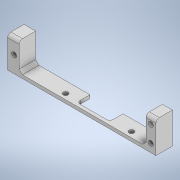
# Autodesk Inventor part: atx-adapter_mount
Saved by Autodesk Inventor 2021 (Build 250183000, 183)
## iProperties
Created: 2024-03-17
Part Number: atx-adapter_mount
Material: Generic
Document SubType Name: Modeling
Designer: Toby
Density: 1 g/cm^3
Appearance: Default
Author: Toby
Autodesk Inventor part; units mm, degrees
ref_plane "YZ Plane" through (0, 0, 0) normal (1, 0, 0) x (0, 1, 0)
ref_plane "XZ Plane" through (0, 0, 0) normal (0, 1, 0) x (-1, 0, 0)
ref_plane "XY Plane" through (0, 0, 0) normal (0, 0, 1) x (1, 0, 0)
sketch "Sketch1" plane through (0, 0, 0) normal (0, 0, 1) x (1, 0, 0)
  line L0 (-40.9154, -1.8235) -> (49.0846, -1.8235)
  line L1 (49.0846, -1.8235) -> (49.0846, -3.8235)
  line L2 (49.0846, -3.8235) -> (-40.9154, -3.8235)
  line L3 (-40.9154, -3.8235) -> (-40.9154, -1.8235)
  line L4 (-40.9154, -1.8235) -> (-33.9154, -1.8235)
  line L5 (-33.9154, -1.8235) -> (-33.9154, 15.1765)
  line L6 (-33.9154, 15.1765) -> (-40.9154, 15.1765)
  line L7 (-40.9154, 15.1765) -> (-40.9154, -1.8235)
  line L8 (49.0846, -1.8235) -> (43.0846, -1.8235)
  line L9 (43.0846, -1.8235) -> (43.0846, 15.1765)
  line L10 (43.0846, 15.1765) -> (49.0846, 15.1765)
  line L11 (49.0846, 15.1765) -> (49.0846, -1.8235)
  circle A0 centre (-36.9154, 6.1765) radius 1.5
  circle A1 centre (46.0846, 11.1765) radius 1.5
  circle A2 centre (46.0846, 1.1765) radius 1.5
  point P0 (0, 0)
  point P1 (43.0846, -1.8235)
  point P2 (43.0846, -1.8235)
  dimension "d0" = 2
  dimension "d1" = 90
  dimension "d2" = 10
  dimension "d3" = 5
  dimension "d4" = 15
  dimension "d5" = 83
  dimension "d6" = 83
  dimension "d7" = 4
  dimension "d8" = 3
  dimension "d9" = 3
  dimension "d10" = 3
  dimension "d11" = 19
  dimension "d12" = 3
  dimension "d13" = 3
  dimension "d14" = 3
  constraints: 24 end point, 6 parallel, 3 centre point, 3 coincident, 3 horizontal, 3 perpendicular, 1 point on line
  measures "d0" distance between parallel lines of L2 L0
  measures "d1" distance of L0.start L0.end
  measures "d2" distance from line of L2 point (-36.915, 6.177)
  measures "d3" distance from line of L2 point (46.085, 1.177)
  measures "d4" distance from line of L2 point (46.085, 11.177)
  measures "d5" horizontal distance of point (-36.915, 6.177) point (46.085, 11.177)
  measures "d6" horizontal distance of point (-36.915, 6.177) point (46.085, 1.177)
  measures "d7" distance from line of L7 point (-36.915, 6.177)
  measures "d8" distance from line of point (-36.915, 6.177) L5
  measures "d9" distance from line of point (46.085, 1.177) L9
  measures "d10" distance from line of point (46.085, 1.177) L11
  measures "d11" distance between parallel lines of L2 L10
  measures "d12" diameter of A0
  measures "d13" diameter of A1
  measures "d14" diameter of A2
extrude "Extrusion1" add sketch "Sketch1" against normal blind 10 contours L7 L6 L5 L0 | L0 L1 L2 L3 | L9 L10 L11 L0 | A0 | A1 | A2
fillet "Fillet1" radius 2 2 edges at (-37.4154, 15.1765, 0) (46.0846, 15.1765, 0)
sketch "Sketch2" plane through (0, 0, 0) normal (0, 0, 1) x (1, 0, 0)
  line L0 (-40.9154, -3.8235) -> (49.0846, -3.8235) projected
  line L1 (-40.9154, 13.1765) -> (-40.9154, -3.8235) projected
  line L2 (49.0846, -3.8235) -> (49.0846, 13.1765) projected
  point P0 (0, 0)
  point P1 (-36.9154, 6.1765)
  point P2 (46.0846, 1.1765)
  point P3 (46.0846, 11.1765)
  dimension "d18" = 10
  dimension "d19" = 5
  dimension "d20" = 15
  dimension "d21" = 4
  dimension "d22" = 83
  dimension "d23" = 83
  dimension "d24" = 3
  measures "d18" distance from line of L0 point (-36.915, 6.177)
  measures "d19" distance from line of L0 point (46.085, 1.177)
  measures "d20" distance from line of L0 point (46.085, 11.177)
  measures "d21" distance from line of L1 point (-36.915, 6.177)
  measures "d22" horizontal distance of point (46.085, 11.177) point (-36.915, 6.177)
  measures "d23" horizontal distance of point (-36.915, 6.177) point (46.085, 1.177)
  measures "d24" distance from line of L2 point (46.085, 1.177)
hole "Hole1" at (-36.9154, 6.1765, 0) at (46.0846, 1.1765, 0) at (46.0846, 11.1765, 0) direction (0, 0, -1) diameter 3 depth 10 tip angle 118
chamfer "Chamfer1" distance 2 angle 45 2 edges at (-33.9154, -1.8235, -5) (43.0846, -1.8235, -5)
sketch "Sketch3" plane through (-31.9154, -1.8235, 0) normal (0, 1, 0) x (1, 0, 0)
  line L0 (73, 0) -> (0, 0) projected
  line L1 (73, 10) -> (73, 0) projected
  point P0 (31.9154, 0)
  point P1 (23, 3.2)
  point P2 (63, 3.2)
  point P3 (68.374, 17.0038)
  dimension "d35" = 3.2
  dimension "d36" = 3.2
  dimension "d37" = 10
  dimension "d38" = 50
  measures "d35" distance from line of L0 point (63, 3.2)
  measures "d36" distance from line of L0 point (23, 3.2)
  measures "d37" distance from line of L1 point (63, 3.2)
  measures "d38" distance from line of L1 point (23, 3.2)
hole "Hole2" at (-8.9154, -1.8235, -3.2) at (31.0846, -1.8235, -3.2) at (36.4586, -1.8235, -17.0038) direction (0, -1, 0) diameter 3 depth 10 tip angle 118
sketch "Sketch4" plane through (-31.9154, -1.8235, 0) normal (0, 1, 0) x (1, 0, 0)
  line L0 (0, 10) -> (73, 10) projected
  line L1 (31, 10) -> (51, 10)
  line L2 (51, 10) -> (51, 2)
  line L3 (51, 2) -> (31, 2)
  line L4 (31, 2) -> (31, 10)
  circle A0 centre (23, 3.2) radius 1.5 projected
  circle A1 centre (63, 3.2) radius 1.5 projected
  line L5 (73, 0) -> (0, 0) projected
  point P0 (31.9154, 0)
  dimension "d46" = 8
  dimension "d47" = 12
  dimension "d48" = 2
  constraints: 8 end point, 2 parallel, 1 horizontal, 1 perpendicular, 1 point on line
  measures "d46" distance from line of A0.centre L4
  measures "d47" distance from line of L2 A1.centre
  measures "d48" distance between parallel lines of L5 L3
extrude "Extrusion2" cut sketch "Sketch4" against normal blind 2 contours L0 L2 L3 L4
fillet "Fillet2" radius 2 2 edges at (-0.9154, -2.8235, -2) (19.0846, -2.8235, -2)
body "Solid1"
